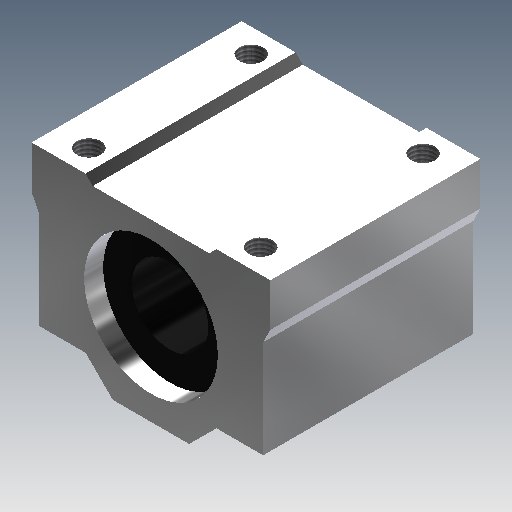
# Autodesk Inventor part: SC16
Saved by Autodesk Inventor 2017 (Build 210142000, 142)
## iProperties
Company: Selvox Ltd.
Created: 2016-03-15
Part Number: SC16
Material: Алюминий 6061
Document SubType Name: Modeling
Designer: Stan Khalipa
Density: 2.7 g/cm^3
Appearance: Алюминий — плоский
Catalog Web Link: http://purelogic.ru
Vendor: Purelogic R&D
Description: Модуль с подшипником серии SC 16мм
Mass: 158.309 g
Surface Area: 140.273 cm^2
Volume: 58.6331 cm^3
Author: Stan Khalipa
Autodesk Inventor part; units mm, degrees
ref_plane "YZ Plane" through (0, 0, 0) normal (1, 0, 0) x (0, 1, 0)
ref_plane "XZ Plane" through (0, 0, 0) normal (0, 1, 0) x (-1, 0, 0)
ref_plane "XY Plane" through (0, 0, 0) normal (0, 0, 1) x (1, 0, 0)
sketch "Эскиз1" plane through (0, 0, 0) normal (0, 0, 1) x (1, 0, 0)
  line L0 (8, -19.1) -> (-8, -19.1)
  line L1 (-23.5, 7.1) -> (-23.5, -13.4)
  line L2 (23.5, 7.1) -> (23.5, -13.4)
  circle A0 centre (0, 0) radius 8
  line L3 (8, -19.1) -> (13.7, -13.4)
  line L4 (-8, -19.1) -> (-13.7, -13.4)
  line L5 (-25, 10.1) -> (-23.5, 7.1)
  line L6 (25, 10.1) -> (23.5, 7.1)
  line L7 (-12.2, 17.6) -> (12.2, 17.6)
  line L8 (-13.7, 19.1) -> (-12.2, 17.6)
  line L9 (13.7, 19.1) -> (12.2, 17.6)
  line L10 (-25, 10.1) -> (-25, 19.1)
  line L11 (25, 19.1) -> (25, 10.1)
  line L12 (-23.5, -13.4) -> (-13.7, -13.4)
  line L13 (13.7, -13.4) -> (23.5, -13.4)
  line L14 (-25, 19.1) -> (-13.7, 19.1)
  line L15 (13.7, 19.1) -> (25, 19.1)
  dimension "d14" = 16
  dimension "d15" = 38.2
  dimension "d16" = 50
  dimension "d17" = 47
  dimension "d18" = 32.5
  dimension "d19" = 2.1213
  dimension "d20" = 135
  dimension "d21" = 24.4
  dimension "d22" = 16
  dimension "d23" = 135
  dimension "d24" = 9.8
  dimension "d25" = 20.5
  dimension "d26" = 9
  dimension "d27" = 9
  dimension "d28" = 11.3
  dimension "d29" = 23.5
  dimension "d30" = 17.6
  dimension "d31" = 3
  constraints: 32 end point, 8 horizontal alignment, 7 perpendicular, 6 vertical alignment, 3 parallel, 2 horizontal, 1 centre point, 1 coincident
  measures "d14" diameter of A0
  measures "d15" distance between parallel lines of L0 L14
  measures "d16" distance between parallel lines of L11 L10
  measures "d17" distance between parallel lines of L2 L1
  measures "d18" distance between parallel lines of L13 L15
  measures "d19" distance of L8.start L7.start
  measures "d20" angle of L8 L14
  measures "d21" distance of L7.start L7.end
  measures "d22" distance of L0.start L0.end
  measures "d23" angle of L13 L3
  measures "d24" distance of L4.end L1.end
  measures "d25" distance of L1.end L1.start
  measures "d26" distance of L5.start L10.end
  measures "d27" distance of L6.start L11.start
  measures "d28" distance of L11.start L9.start
  measures "d29" distance from line of L1 point (0, 0)
  measures "d30" distance from line of point (0, 0) L7
  measures "d31" vertical distance of L2.start L6.start
extrude "Выдавливание1" add sketch "Эскиз1" along normal mid plane 44
sketch "Эскиз2" plane through (-25, 19.1, 22) normal (0, 1, 0) x (1, 0, 0)
  circle A0 centre (7, 39) radius 2.5
  circle A1 centre (7, 5) radius 2.5
  circle A2 centre (43, 39) radius 2.5
  circle A3 centre (43, 5) radius 2.5
  line L0 (0, 0) -> (0, 44) projected
  line L1 (0, 44) -> (11.3, 44) projected
  point P0 (25, 22)
  dimension "d34" = 5
  dimension "d39" = 5
  dimension "d40" = 5
  dimension "d41" = 5
  dimension "d42" = 36
  dimension "d43" = 34
  dimension "d44" = 7
  dimension "d45" = 5
  constraints: 4 centre point, 2 horizontal alignment, 2 vertical alignment
  measures "d34" diameter of A0
  measures "d39" diameter of A1
  measures "d40" diameter of A2
  measures "d41" diameter of A3
  measures "d42" distance of A3.centre A1.centre
  measures "d43" distance of A1.centre A0.centre
  measures "d44" distance from line of A0.centre L0
  measures "d45" distance from line of L1 A0.centre
hole "Отверстие1" at (-18, 19.1, 17) at (-18, 19.1, -17) at (18, 19.1, -17) at (18, 19.1, 17) direction (0, -1, 0) diameter 5 depth 19 tip angle 118
thread "Резьба1" size "M5x0.8" class "6H" standard "ANSI Metric M Profile" full length
thread "Резьба2" size "M5x0.8" class "6H" standard "ANSI Metric M Profile" full length
thread "Резьба3" size "M5x0.8" class "6H" standard "ANSI Metric M Profile" full length
thread "Резьба4" size "M5x0.8" class "6H" standard "ANSI Metric M Profile" full length
sketch "Эскиз3" plane through (0, 0, 22) normal (0, 0, 1) x (1, 0, 0)
  circle A0 centre (0, 0) radius 14
  dimension "d61" = 28
  constraints: 1 centre point, 1 coincident
  measures "d61" diameter of A0
extrude "Выдавливание2" cut sketch "Эскиз3" against normal blind 4
sketch "Эскиз4" plane through (0, 0, -22) normal (0, 0, -1) x (-1, 0, 0)
  circle A0 centre (0, 0) radius 14
  dimension "d64" = 28
  constraints: 1 centre point, 1 coincident
  measures "d64" diameter of A0
extrude "Выдавливание3" cut sketch "Эскиз4" against normal blind 4
sketch "Sketch5" plane through (-25, 19.1, 22) normal (0, 1, 0) x (1, 0, 0)
  point P0 (7, 39)
  point P1 (43, -92)
  point P2 (7, -92)
  point P3 (-62, 39)
  point P4 (-98, 39)
  point P5 (-98, -92)
  point P6 (-98, -58)
  point P7 (-62, -92)
  point P8 (-62, -58)
  point P9 (-98, 5)
  point P10 (-62, 5)
  point P11 (43, 39)
